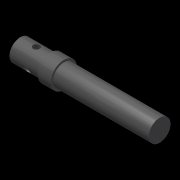
# Autodesk Inventor part: Ball Shift
Saved by Autodesk Inventor 2014 SP1 (Build 180222100, 222)
## iProperties
Created: 2014-01-20
Part Number: Ball Shift
Material: Generic
Document SubType Name: Modeling
Designer: Rauhul Varma
Density: 1 g/cm^3
Appearance: Steel
Mass: 18.6658 g
Surface Area: 64.4337 cm^2
Volume: 18.6658 cm^3
Author: Rauhul Varma
Autodesk Inventor part; units mm, degrees
ref_plane "YZ Plane" through (0, 0, 0) normal (1, 0, 0) x (0, 1, 0)
ref_plane "XZ Plane" through (0, 0, 0) normal (0, 1, 0) x (-1, 0, 0)
ref_plane "XY Plane" through (0, 0, 0) normal (0, 0, 1) x (1, 0, 0)
sketch "Sketch1" plane through (0, 0, 0) normal (0, 0, 1) x (1, 0, 0)
  line L0 (0, 0) -> (21.9725, 0)
  line L1 (40.4812, 0) -> (40.4812, 7.9375) construction
  line L2 (40.4812, 7.9375) -> (31.75, 7.9375)
  line L3 (0, 7.9375) -> (0, 6.35)
  line L4 (31.75, 0) -> (31.75, 7.9375) construction
  line L5 (31.75, 9.525) -> (22.225, 9.525)
  line L6 (22.225, 9.525) -> (22.225, 7.9375)
  line L7 (8.7312, 0) -> (8.7312, 17.4625) construction
  line L8 (8.7312, 17.4625) -> (0, 17.4625) construction
  line L9 (0, 17.4625) -> (0, 7.9375) construction
  line L10 (8.7312, 14.2875) -> (9.525, 14.2875) construction
  line L11 (9.525, 14.2875) -> (9.525, 7.9375) construction
  line L12 (9.525, 14.2875) -> (9.525, 27.94) construction
  line L13 (9.525, 27.94) -> (19.05, 27.94) construction
  line L14 (19.05, 27.94) -> (19.05, 7.9375) construction
  line L15 (22.225, 9.525) -> (22.225, 14.2875) construction
  line L16 (22.225, 14.2875) -> (21.4312, 14.2875) construction
  line L17 (21.4312, 14.2875) -> (21.4312, 7.9375) construction
  line L18 (21.4312, 14.2875) -> (21.4312, 17.4625) construction
  line L19 (21.4312, 17.4625) -> (14.2875, 17.4625) construction
  line L20 (14.2875, 17.4625) -> (14.2875, 0) construction
  line L21 (14.2875, 27.94) -> (14.2875, 17.4625) construction
  line L22 (14.1605, 27.94) -> (14.1605, 0) construction
  line L23 (11.9062, 27.94) -> (11.9062, 0) construction
  circle A0 centre (11.9062, 7.5565) radius 2.3813 construction
  line L24 (0, 5.5562) -> (6.2514, 5.5563) construction
  line L25 (0, 6.35) -> (6.2514, 6.35)
  line L26 (6.2514, 6.35) -> (6.2514, 5.5563)
  line L27 (6.2514, 5.5563) -> (6.2514, 0) construction
  line L28 (9.8391, 5.1753) -> (13.9734, 5.1753) construction
  line L29 (0, 3.175) -> (12.7284, 3.175)
  line L30 (6.2514, 5.5563) -> (19.0308, 5.5563)
  line L31 (0, 6.35) -> (0, 0) construction
  circle A1 centre (11.9062, 5.5562) radius 2.3813 construction
  circle A2 centre (11.9062, 5.8103) radius 2.3813 construction
  line L32 (14.2875, 8.1915) -> (9.525, 8.1915) construction
  line L33 (0, 3.175) -> (-5.4674, 3.175)
  line L34 (-5.4674, 3.175) -> (-5.4674, 2.3813)
  line L35 (-5.4674, 2.3813) -> (-10.4458, 2.3812)
  line L36 (-10.4458, 2.3812) -> (-10.4458, 0)
  line L37 (-10.4458, 0) -> (0, 0)
  line L38 (9.8391, 5.1753) -> (7.8389, 3.175) construction
  line L39 (12.7284, 3.175) -> (14.7286, 5.1753)
  line L40 (13.9734, 5.1753) -> (17.083, 0) construction
  line L41 (14.7286, 5.1753) -> (18.8629, 5.1753)
  line L42 (18.8629, 5.1753) -> (21.9725, 0)
  line L43 (19.0308, 5.5563) -> (22.3693, 0)
  line L44 (22.225, 5.5563) -> (31.75, 5.5563) construction
  line L45 (19.0308, 5.5563) -> (22.225, 5.5563) construction
  line L46 (22.225, 7.9375) -> (22.225, 0) construction
  line L47 (31.75, 7.9375) -> (31.75, 9.525)
  line L48 (31.75, 7.9375) -> (22.225, 7.9375) construction
  line L49 (22.225, 7.9375) -> (0, 7.9375)
  line L50 (31.75, 5.5563) -> (40.4812, 5.5563) construction
  line L51 (22.225, 0) -> (22.3693, 0) construction
  line L52 (22.3693, 0) -> (22.225, 0) construction
  line L53 (21.9725, 0) -> (22.3693, 0) construction
  line L54 (12.7284, 3.175) -> (40.4812, 3.175) construction
  line L55 (40.4812, 7.9375) -> (101.6, 7.9375)
  line L56 (101.6, 7.9375) -> (101.6, 0)
  line L57 (101.6, 0) -> (40.4812, 0)
  line L58 (22.3693, 0) -> (40.4812, 0)
  dimension "d0" = 7.9375
  dimension "d1" = 40.4813
  dimension "d2" = 9.525
  dimension "d3" = 8.7312
  dimension "d5" = 22.225
  dimension "d6" = 17.4625
  dimension "d7" = 8.7312
  dimension "d8" = 0.7937
  dimension "d9" = 14.2875
  dimension "d10" = 27.94
  dimension "d11" = 9.525
  dimension "d12" = 0.7937
  dimension "d14" = 7.1437
  dimension "d15" = 17.4625
  dimension "d16" = 0.127
  dimension "d17" = 4.7625
  dimension "d18" = 4.7625
  dimension "d19" = 5.5563
  dimension "d20" = 6.35
  dimension "d22" = 3.175
  dimension "d23" = 4.7625
  dimension "d24" = 4.7625
  dimension "d25" = 4.7625
  dimension "d26" = 0.254
  dimension "d27" = 2.0671
  dimension "d29" = 0.381
  dimension "d30" = 5.4673
  dimension "d31" = 4.9784
  dimension "d32" = 2.3813
  dimension "d33" = 45
  dimension "d34" = 45
  dimension "d35" = 0.0635
  dimension "d36" = 2.0671
  dimension "d37" = 59
  dimension "d38" = 4.1342
  dimension "d39" = 1.5875
  dimension "d40" = 0.3969
  dimension "d41" = 9.525
  dimension "d42" = 14.2875
  dimension "d43" = 61.1187
  dimension "d45" = 14.7287
  dimension "d46" = 9.8392
  constraints: 116 end point, 63 perpendicular, 29 point on line, 28 parallel, 7 horizontal, 7 vertical, 4 tangent, 3 centre point, 2 collinear, 2 midpoint, 10 other
  measures "d0" distance of L3.start L31.end
  measures "d1" distance of L1.end L3.start
  measures "d2" distance between parallel lines of L4 L6
  measures "d3" distance between parallel lines of L1 L4
  measures "d5" distance between parallel lines of L3 L6
  measures "d6" distance of the line from the sketch origin of L8
  measures "d7" distance of L7.end L8.end
  measures "d8" distance between parallel lines of L7 L11
  measures "d9" distance of the line from the sketch origin of L10
  measures "d10" distance of the line from the sketch origin of L13
  measures "d11" distance of L12.end L13.end
  measures "d12" distance between parallel lines of L15 L17
  measures "d14" distance of L18.end L19.end
  measures "d15" distance of the line from the sketch origin of L19
  measures "d16" distance between parallel lines of L22 L20
  measures "d17" diameter of L12 L23
  measures "d18" diameter of A0
  measures "d19" distance of the line from the sketch origin of L24
  measures "d20" distance of the line from the sketch origin of L25
  measures "d22" distance of the line from the sketch origin of L29
  measures "d23" diameter of A1
  measures "d24" diameter of A2
  measures "d25" distance of L32.start L32.end
  measures "d26" distance between parallel lines of L2 L32
  measures "d27" distance from line of L23 L28.start
  measures "d29" distance between parallel lines of L30 L28
  measures "d30" distance of L29.start L33.end
  measures "d31" distance of L34.end L35.end
  measures "d32" distance of the line from the sketch origin of L35
  measures "d33" angle of L29 L38
  measures "d34" angle of L29 L39
  measures "d35" distance edge to line of A2 L39
  measures "d36" distance from line of L23 L28.end
  measures "d37" angle to the sketch x axis of L40
  measures "d38" distance of L39.end L41.end
  measures "d39" distance from line of L27 L38.end
  measures "d40" distance of L43.end L42.end
  measures "d41" distance between parallel lines of L51 L5
  measures "d42" distance of the line from the sketch origin of L16
  measures "d43" distance of L1.end L55.end
  measures "d45" distance from line of L31 L39.end
  measures "d46" distance from line of L31 L28.start
revolve "Revolution1" add sketch "Sketch1" angle 360 about axis through (101.6, 0, 0) along (-1, 0, 0) contours L55 L56 L57 L58 L43 L30 L26 L25 L3 L49 L6 L5 L47 L2
sketch "Sketch2" plane through (0, 0, 0) normal (0, 1, 0) x (-1, 0, 0)
  point P0 (0, 0)
  point P1 (-11.9062, 0)
  point P2 (-11.9062, 0)
  point P3 (-11.9062, 0)
  point P4 (-11.9062, 0)
  constraints: 1 coincident
hole "Hole1" at (11.9062, 0, 0) direction (0, 1, 0) diameter 4.8514 end through all
pattern_circular "Circular Pattern1" count 3 over 360 about axis through (-10, 0, 0) along (1, 0, 0) of "Hole1"
equation "\"d7\" = d3"
equation "\"d12\" = d8"
equation "\"d15\" = d6"
equation "\"d34\" = d33"
equation "\"d36\" = d27"
equation "\"d38\" = d27 + d36"
equation "\"d42\" = d9"
body "Solid1"
